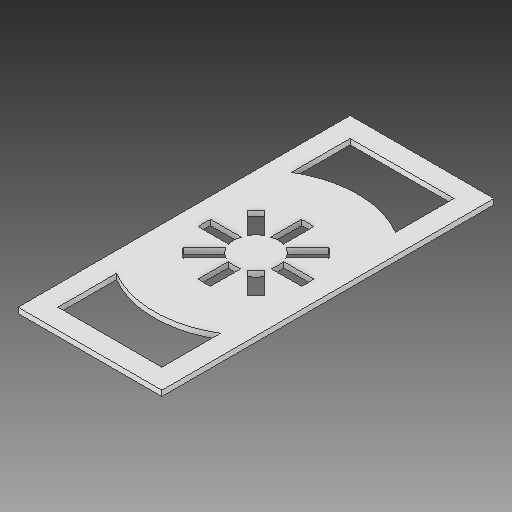
# Autodesk Inventor part: Cuerpo - Base
Saved by Autodesk Inventor 2019 (Build 230136000, 136)
## iProperties
Created: 2020-02-15
Part Number: Cuerpo - Base
Material: ABS Plastic
Document SubType Name: Modeling
Designer: Mafer1
Density: 1.06 g/cm^3
Appearance: Smooth - White
Mass: 43.8755 g
Surface Area: 296.565 cm^2
Volume: 41.392 cm^3
ancho_base: 80.000 mm
largo_base: 200.000 mm
Author: Mafer1
Autodesk Inventor part; units mm, degrees
ref_plane "YZ Plane" through (0, 0, 0) normal (1, 0, 0) x (0, 1, 0)
ref_plane "XZ Plane" through (0, 0, 0) normal (0, 1, 0) x (-1, 0, 0)
ref_plane "XY Plane" through (0, 0, 0) normal (0, 0, 1) x (1, 0, 0)
sketch "Boceto1" plane through (0, 0, 0) normal (0, 1, 0) x (-1, 0, 0)
  line L0 (0, 0) -> (86.6, 0)
  line L1 (86.6, 0) -> (86.6, -200)
  line L2 (86.6, -200) -> (0, -200)
  line L3 (0, -200) -> (0, 0)
  dimension "d0" = 200
  dimension "d1" = 86.6
  constraints: 8 end point, 2 parallel, 1 horizontal, 1 perpendicular
  measures "d0" distance of L0.end L1.end
  measures "d1" distance between parallel lines of L3 L1
extrude "Extrusión1" add sketch "Boceto1" along normal blind 3.3
sketch "Boceto2" plane through (0, 3.3, 0) normal (0, 1, 0) x (1, 0, 0)
  circle A0 centre (-43.3, 100) radius 13.3 construction
  circle A1 centre (-43.3, 100) radius 31.3 construction
  line L0 (-74.6, 152.7067) -> (-74.6, 188)
  line L1 (-74.6, 188) -> (-12, 188)
  line L2 (-12, 188) -> (-12, 152.7067)
  line L3 (-74.6, 47.2933) -> (-74.6, 12)
  line L4 (-74.6, 12) -> (-12, 12)
  line L5 (-12, 12) -> (-12, 47.2933)
  arc A2 (-12, 152.7067) -> (-74.6, 152.7067) centre (-43.3, 100) ccw
  arc A3 (-74.6, 47.2933) -> (-12, 47.2933) centre (-43.3, 100) ccw
  line L6 (-86.6, 0) -> (0, 0) projected
  line L7 (0, 0) -> (0, 200) projected
  line L8 (0, 200) -> (-86.6, 200) projected
  line L9 (-86.6, 200) -> (-86.6, 0) projected
  line L10 (0, 200) -> (-86.6, 200) projected
  line L11 (-47.05, 68.9255) -> (-47.05, 87.2396)
  line L12 (-39.55, 68.9255) -> (-39.55, 87.2396)
  arc A4 (-47.05, 87.2396) -> (-39.55, 87.2396) centre (-43.3, 100) ccw
  arc A5 (-47.05, 68.9255) -> (-39.55, 68.9255) centre (-43.3, 100) ccw
  line L13 (-18.6753, 80.6786) -> (-31.6254, 93.6287)
  arc A6 (-23.9786, 75.3753) -> (-18.6753, 80.6786) centre (-43.3, 100) ccw
  line L14 (-23.9786, 75.3753) -> (-36.9287, 88.3254)
  arc A7 (-36.9287, 88.3254) -> (-31.6254, 93.6287) centre (-43.3, 100) ccw
  line L15 (-12.2255, 103.75) -> (-30.5396, 103.75)
  arc A8 (-12.2255, 96.25) -> (-12.2255, 103.75) centre (-43.3, 100) ccw
  line L16 (-12.2255, 96.25) -> (-30.5396, 96.25)
  arc A9 (-30.5396, 96.25) -> (-30.5396, 103.75) centre (-43.3, 100) ccw
  line L17 (-23.9786, 124.6247) -> (-36.9287, 111.6746)
  arc A10 (-18.6753, 119.3214) -> (-23.9786, 124.6247) centre (-43.3, 100) ccw
  line L18 (-18.6753, 119.3214) -> (-31.6254, 106.3713)
  arc A11 (-31.6254, 106.3713) -> (-36.9287, 111.6746) centre (-43.3, 100) ccw
  line L19 (-47.05, 131.0745) -> (-47.05, 112.7604)
  arc A12 (-39.55, 131.0745) -> (-47.05, 131.0745) centre (-43.3, 100) ccw
  line L20 (-39.55, 131.0745) -> (-39.55, 112.7604)
  arc A13 (-39.55, 112.7604) -> (-47.05, 112.7604) centre (-43.3, 100) ccw
  line L21 (-67.9247, 119.3214) -> (-54.9746, 106.3713)
  arc A14 (-62.6214, 124.6247) -> (-67.9247, 119.3214) centre (-43.3, 100) ccw
  line L22 (-62.6214, 124.6247) -> (-49.6713, 111.6746)
  arc A15 (-49.6713, 111.6746) -> (-54.9746, 106.3713) centre (-43.3, 100) ccw
  line L23 (-74.3745, 96.25) -> (-56.0604, 96.25)
  arc A16 (-74.3745, 103.75) -> (-74.3745, 96.25) centre (-43.3, 100) ccw
  line L24 (-74.3745, 103.75) -> (-56.0604, 103.75)
  arc A17 (-56.0604, 103.75) -> (-56.0604, 96.25) centre (-43.3, 100) ccw
  line L25 (-62.6214, 75.3753) -> (-49.6713, 88.3254)
  arc A18 (-67.9247, 80.6786) -> (-62.6214, 75.3753) centre (-43.3, 100) ccw
  line L26 (-67.9247, 80.6786) -> (-54.9746, 93.6287)
  arc A19 (-54.9746, 93.6287) -> (-49.6713, 88.3254) centre (-43.3, 100) ccw
  line L27 (-86.6, 200) -> (-86.6, 0) projected
  line L28 (0, 0) -> (0, 200) projected
  point P0 (-43.3, 200)
  point P1 (-86.6, 100)
  point P2 (-43.3, 200)
  point P3 (-43.3, 86.7)
  point P4 (-33.8955, 90.5955)
  point P5 (-30, 100)
  point P6 (-33.8955, 109.4045)
  point P7 (-43.3, 113.3)
  point P8 (-52.7045, 109.4045)
  point P9 (-56.6, 100)
  point P10 (-52.7045, 90.5955)
  dimension "d4" = 12
  dimension "d5" = 12
  dimension "d6" = 12
  dimension "d7" = 12
  dimension "d8" = 30
  dimension "d9" = 30
  dimension "d10" = 18
  dimension "d11" = 7.5
  dimension "d14" = 360
  dimension "d19" = 30
  constraints: 44 end point, 41 point on circle, 20 centre point, 4 concentric, 4 perpendicular, 3 midpoint, 3 parallel, 3 vertical, 3 vertical alignment, 2 point on line, 1 coincident, 1 collinear, 1 horizontal alignment, 89 other
  measures "d4" distance between parallel lines of L8 L1
  measures "d5" distance between parallel lines of L9 L0
  measures "d6" distance between parallel lines of L7 L2
  measures "d7" distance between parallel lines of L6 L4
  measures "d8" radial gap between concentric circles of A3 A1
  measures "d9" radial gap between concentric circles of A1 A2
  measures "d10" radial gap between concentric circles of A1 A0
  measures "d11" distance between parallel lines of L12 L11
  measures "d19" distance of point (-86.6, 100) point (-56.6, 100)
extrude "Extrusión2" cut sketch "Boceto2" against normal blind 10 contours L0 L1 L2 A2 | A3 L5 L4 L3 | L11 A4 L12 A5 | A6 L14 A7 L13 | A8 L16 A9 L15 | A10 L18 A11 L17 | A12 L20 A13 L19 | A14 L22 A15 L21 | A16 L24 A17 L23 | A18 L26 A19 L25
equation "\"d0\" = largo_base"
equation "\"d5\" = d4"
equation "\"d6\" = d4"
equation "\"d7\" = d4"
equation "\"d9\" = d19"
equation "\"d10\" = 1.5 * d4"
equation "\"d11\" = 0.25 * d19"
equation "\"d19\" = d8"
equation "\"ancho_base\" = 80"
equation "\"largo_base\" = 200"
